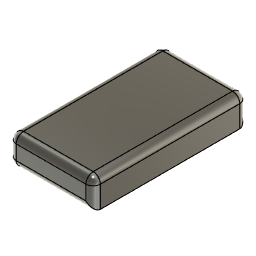
Chassis v11 (Autodesk Fusion 360 archive; units mm, degrees)
design "Battery"
Autodesk Fusion 360 part; units mm, degrees
sketch "Sketch1" plane through (0, 0, 0) normal (0, 0, 1) x (1, 0, 0)
  line L0 (-14.5, 26.5) -> (14.5, 26.5)
  line L1 (14.5, 26.5) -> (14.5, -26.5)
  line L2 (14.5, -26.5) -> (-14.5, -26.5)
  line L3 (-14.5, -26.5) -> (-14.5, 26.5)
  dimension "d1" = 29
  dimension "d2" = 53
  constraint horizontal L0
  constraint vertical L1
  constraint horizontal L2
  constraint vertical L3
  measures "d1" distance of L0.start L0.end
  measures "d2" distance of L0.start L2.end
extrude "Extrude1" add sketch "Sketch1" along normal blind 10
fillet "Fillet1" radius 2.5 9 edges at (-14.5, -26.5, 5) (0, 26.5, 10) (-14.5, 26.5, 5) (0, 26.5, 0) (14.5, 0, 10) (0, -26.5, 10) (-14.5, 0, 0) (-14.5, 0, 10) (14.5, 26.5, 5) 4 faces at (4.8333, -26.5, 3.3333) (-4.8333, 26.5, 3.3333) (-4.8333, -8.8333, 10) (-14.5, -8.8333, 3.3333)
